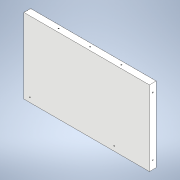
# Autodesk Inventor part: Tapa_superior_izquierda
Saved by Autodesk Inventor 2021 (Build 250183000, 183)
## iProperties
Created: 2021-04-15
Part Number: Tapa_superior_izquierda
Material: Genérico
Document SubType Name: Modeling
Designer: Admin
Density: 1 g/cm^3
Appearance: Blanco
Author: Admin
Autodesk Inventor part; units mm, degrees
ref_plane "YZ Plane" through (0, 0, 0) normal (1, 0, 0) x (0, 1, 0)
ref_plane "XZ Plane" through (0, 0, 0) normal (0, 1, 0) x (-1, 0, 0)
ref_plane "XY Plane" through (0, 0, 0) normal (0, 0, 1) x (1, 0, 0)
sketch "Boceto1" plane through (0, 0, 0) normal (0, 0, 1) x (1, 0, 0)
  line L0 (0, 0) -> (385, 0)
  line L1 (385, 0) -> (385, 230)
  line L2 (385, 230) -> (0, 230)
  line L3 (0, 230) -> (0, 0)
  dimension "d0" = 385
  dimension "d1" = 230
  constraints: 8 end point, 2 parallel, 1 horizontal, 1 perpendicular
  measures "d0" distance of L2.end L1.end
  measures "d1" distance of L1.end L0.end
extrude "Extrusión1" add sketch "Boceto1" along normal blind 0.76
sketch "Boceto2" plane through (0, 0, 0.76) normal (0, 0, 1) x (1, 0, 0)
  line L0 (385, 230) -> (0, 230) projected
  line L1 (0, 0) -> (0.76, 0)
  line L2 (0.76, 0.76) -> (0.76, 229.24)
  line L3 (0.76, 230) -> (0, 230)
  line L4 (0, 230) -> (0, 0)
  line L5 (0, 230) -> (0, 0) projected
  line L6 (385, 0) -> (385, 230) projected
  line L7 (0, 0) -> (385, 0)
  line L8 (385, 0) -> (385, 0.76)
  line L9 (384.24, 0.76) -> (0.76, 0.76)
  line L10 (0, 0.76) -> (0, 0)
  line L11 (0, 0) -> (385, 0) projected
  line L12 (385, 0) -> (384.24, 0)
  line L13 (384.24, 0.76) -> (384.24, 229.24)
  line L14 (384.24, 230) -> (385, 230)
  line L15 (385, 230) -> (385, 0)
  line L16 (385, 230) -> (0, 230)
  line L17 (0, 230) -> (0, 229.24)
  line L18 (0.76, 229.24) -> (384.24, 229.24)
  line L19 (385, 229.24) -> (385, 230)
  dimension "d4" = 0.76
  dimension "d5" = 0.76
  dimension "d6" = 0.76
  dimension "d7" = 0.76
  constraints: 32 end point, 8 parallel, 4 horizontal, 4 perpendicular, 4 point on line
  measures "d4" distance of L3.end L3.start
  measures "d5" distance of L8.end L7.end
  measures "d6" distance of L14.start L14.end
  measures "d7" distance of L17.end L16.end
extrude "Extrusión2" add sketch "Boceto2" along normal blind 20
sketch "Boceto3" plane through (0, 0, 0) normal (0, 0, -1) x (-1, 0, 0)
  line L0 (-385, 0) -> (-385, 230) projected
  line L1 (-385, 0) -> (-366, 0)
  line L2 (0, 0) -> (-385, 0) projected
  line L3 (-366, 0) -> (-366, 14)
  circle A0 centre (-366, 14) radius 1.5875
  line L4 (-366, 14) -> (-108, 14)
  circle A1 centre (-108, 14) radius 1.5875
  dimension "d10" = 19
  dimension "d11" = 14
  dimension "d12" = 3.175
  dimension "d13" = 258
  dimension "d14" = 3.175
  constraints: 6 end point, 2 centre point, 2 coincident, 1 horizontal, 1 point on line, 1 vertical
  measures "d10" distance of L0.start L1.end
  measures "d11" distance of L1.end L3.end
  measures "d12" diameter of A0
  measures "d13" distance of L4.start L4.end
  measures "d14" diameter of A1
extrude "Extrusión3" cut sketch "Boceto3" against normal through all
sketch "Boceto4" plane through (0, 230, 0) normal (0, 1, 0) x (1, 0, 0)
  line L0 (0, 0) -> (0, -20.76) construction
  line L1 (0, -10.38) -> (385, -10.38) construction
  line L2 (385, 0) -> (385, -20.76) construction
  line L3 (0, -10.38) -> (96.25, -10.38) construction
  line L4 (96.25, -10.38) -> (192.5, -10.38) construction
  line L5 (192.5, -10.38) -> (288.75, -10.38) construction
  circle A0 centre (96.25, -10.38) radius 1.5875
  circle A1 centre (192.5, -10.38) radius 1.5875
  circle A2 centre (288.75, -10.38) radius 1.5875
  dimension "d17" = 96.25
  dimension "d18" = 96.25
  dimension "d19" = 96.25
  dimension "d20" = 3.175
  dimension "d21" = 3.175
  dimension "d22" = 3.175
  constraints: 8 end point, 3 centre point, 3 coincident, 3 midpoint, 2 point on line
  measures "d17" distance of L1.start L3.end
  measures "d18" distance of L3.end L4.end
  measures "d19" distance of L4.end L5.end
  measures "d20" diameter of A0
  measures "d21" diameter of A1
  measures "d22" diameter of A2
ref_plane "Plano de trabajo1" through (1.52, 228.48, 0.76) normal (0, -1, 0) x (1, 0, 0)
extrude "Extrusión4" cut sketch "Boceto4" against normal up to surface (1.52 mm away)
sketch "Boceto5" plane through (0, 0, 0) normal (-1, 0, 0) x (0, 0, 1)
  line L0 (8.7925, 230) -> (11.9675, 230) construction
  line L1 (10.38, 230) -> (10.38, 0) construction
  line L2 (0, 0) -> (20.76, 0) construction
  line L3 (10.38, 230) -> (10.38, 204.6) construction
  line L4 (10.38, 0) -> (10.38, 25.4) construction
  circle A0 centre (10.38, 204.6) radius 1.5875
  circle A1 centre (10.38, 25.4) radius 1.5875
  dimension "d25" = 25.4
  dimension "d26" = 25.4
  dimension "d27" = 3.175
  dimension "d28" = 3.175
  constraints: 6 end point, 2 centre point, 2 coincident, 2 midpoint, 2 point on line
  measures "d25" distance of L1.start L3.end
  measures "d26" distance of L1.end L4.end
  measures "d27" diameter of A0
  measures "d28" diameter of A1
ref_plane "Plano de trabajo2" through (1.52, 1.52, 0.76) normal (1, 0, 0) x (0, 1, 0)
extrude "Extrusión5" cut sketch "Boceto5" against normal up to surface (1.52 mm away)
